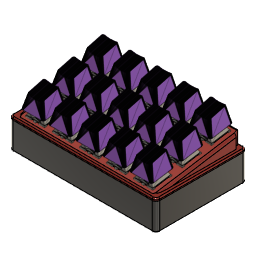
BFDeck x15 v4 (Autodesk Fusion 360 design; units mm, degrees)
Autodesk Fusion 360 part; units mm, degrees
note: some values were not read from the file. Chosen so that the rebuilt part matches the saved one: a direction; which face or edge a step refers to; which pieces of a blend or face edit are solid. Set by a fixed rule: which sketch regions a step uses.
sketch "Sketch1" plane through (0, 0, 0) normal (0, 0, 1) x (1, 0, 0)
  line L0 (-28.1946, -17.8088) -> (89.8054, -17.8088)
  line L1 (89.8054, -17.8088) -> (89.8054, 55.1912)
  line L2 (89.8054, 55.1912) -> (-28.1946, 55.1912)
  line L3 (-28.1946, 55.1912) -> (-28.1946, -17.8088)
  line L4 (87.8054, 53.1912) -> (-26.1946, 53.1912)
  line L5 (-26.1946, 53.1912) -> (-26.1946, -15.8088)
  line L6 (-26.1946, -15.8088) -> (87.8054, -15.8088)
  line L7 (87.8054, -15.8088) -> (87.8054, 53.1912)
  line L8 (87.8054, 53.1912) -> (-26.1946, -15.8088) construction
  line L9 (-26.1946, 53.1912) -> (87.8054, -15.8088) construction
  point P0 (30.8054, 18.6912)
  dimension "d1" = 114
  dimension "d2" = 69
  dimension "d104" = 2
  dimension "d106" = 2
  dimension "d136" = 2
  dimension "d137" = 2
  constraint horizontal L0
  constraint vertical L1
  constraint horizontal L2
  constraint vertical L3
  constraint horizontal L4
  constraint perpendicular L4 L5
  constraint parallel L4 L6
  constraint parallel L5 L7
  constraint coincident L8 P0
  constraint coincident L9 P0
  measures "d1" distance of L5.end L6.end
  measures "d2" distance of L4.end L5.end
  measures "d104" distance of L3 L5
  measures "d106" distance of L0 L6
  measures "d136" distance of L2 L4
  measures "d137" distance of L1 L7
extrude "Extrude1" add sketch "Sketch1" along normal blind 2 contours L0 L1 L2 L3 | L4 L5 L6 L7 makes body 1
sketch "Sketch2" plane through (0, 0, 2) normal (0, 0, 1) x (-1, 0, 0)
  line L0 (28.1946, -55.1912) -> (28.1946, 17.8088)
  line L1 (28.1946, 17.8088) -> (-89.8054, 17.8088)
  line L2 (-89.8054, 17.8088) -> (-89.8054, -55.1912)
  line L3 (-89.8054, -55.1912) -> (28.1946, -55.1912)
  line L4 (-87.8054, -53.1912) -> (26.1946, -53.1912)
  line L5 (26.1946, -53.1912) -> (26.1946, 15.8088)
  line L6 (26.1946, 15.8088) -> (-87.8054, 15.8088)
  line L7 (-87.8054, 15.8088) -> (-87.8054, -53.1912)
  line L8 (-87.8054, -53.1912) -> (26.1946, 15.8088) construction
  line L9 (26.1946, -53.1912) -> (-87.8054, 15.8088) construction
  point P0 (-30.8054, -18.6912)
  dimension "d7" = 114
  dimension "d8" = 69
  dimension "d107" = 2
  dimension "d108" = 2
  constraint horizontal L4
  constraint perpendicular L4 L5
  constraint parallel L4 L6
  constraint parallel L5 L7
  constraint coincident L8 P0
  constraint coincident L9 P0
  measures "d7" distance of L5.end L6.end
  measures "d8" distance of L4.start L6.end
  measures "d107" distance of L3 L4
  measures "d108" distance of L2 L7
extrude "Extrude2" add sketch "Sketch2" along normal blind 20 bodies 1
fillet "Fillet1" radius 3 1 edges at (89.8054, 55.1912, 11) on bodies 1
fillet "Fillet2" radius 3 3 edges at (-28.1946, 55.1912, 11) (-28.1946, -17.8088, 11) (89.8054, -17.8088, 11) on bodies 1
sketch "Sketch3" plane through (0, 0, 2) normal (0, 0, 1) x (-1, 0, 0)
  line L0 (-87.8054, -53.1912) -> (26.1946, -53.1912)
  line L1 (-87.8054, 15.8088) -> (-87.8054, -53.1912)
  line L2 (26.1946, -53.1912) -> (22.1946, -53.1912)
  line L3 (22.1946, -53.1912) -> (22.1946, -52.1912)
  line L4 (25.1946, -49.1912) -> (26.1946, -49.1912)
  line L5 (26.1946, -49.1912) -> (26.1946, -53.1912)
  arc A0 (25.1946, -49.1912) -> (22.1946, -52.1912) centre (25.1946, -52.1912) ccw
  circle A1 centre (25.1946, -52.1912) radius 1
  line L6 (-30.8054, -53.1912) -> (-30.8054, 38.8966)
  line L7 (59.5295, -18.6912) -> (-87.8054, -18.6912)
  line L8 (-87.8054, -49.1912) -> (-87.8054, -53.1912)
  circle A2 centre (-86.8054, -52.1912) radius 1
  arc A3 (-83.8054, -52.1912) -> (-86.8054, -49.1912) centre (-86.8054, -52.1912) ccw
  line L9 (-86.8054, -49.1912) -> (-87.8054, -49.1912)
  line L10 (-87.8054, -53.1912) -> (-83.8054, -53.1912)
  line L11 (-83.8054, -53.1912) -> (-83.8054, -52.1912)
  arc A4 (-86.8054, 11.8088) -> (-83.8054, 14.8088) centre (-86.8054, 14.8088) ccw
  line L12 (-86.8054, 11.8088) -> (-87.8054, 11.8088)
  line L13 (22.1946, 15.8088) -> (22.1946, 14.8088)
  line L14 (-87.8054, 15.8088) -> (26.1946, 15.8088)
  arc A5 (22.1946, 14.8088) -> (25.1946, 11.8088) centre (25.1946, 14.8088) ccw
  line L15 (26.1946, 15.8088) -> (22.1946, 15.8088)
  circle A6 centre (25.1946, 14.8088) radius 1
  line L16 (-83.8054, 15.8088) -> (-83.8054, 14.8088)
  line L17 (26.1946, 11.8088) -> (26.1946, 15.8088)
  line L18 (-87.8054, 11.8088) -> (-87.8054, 15.8088)
  line L19 (25.1946, 11.8088) -> (26.1946, 11.8088)
  circle A7 centre (-86.8054, 14.8088) radius 1
  line L20 (-87.8054, 15.8088) -> (-83.8054, 15.8088)
  line L21 (26.1946, -53.1912) -> (26.1946, 15.8088)
  line L22 (26.1946, 15.8088) -> (-87.8054, 15.8088)
  line L23 (87.2649, 1.901) -> (55, 1.901)
  line L24 (55, 1.901) -> (55, -5)
  line L25 (55, -5) -> (87.2649, -5)
  line L26 (87.2649, -5) -> (87.2649, 1.901)
  point P0 (22.1946, -49.1912)
  point P1 (-83.8054, -49.1912)
  point P2 (-87.8054, -53.1912)
  point P3 (-30.8054, 15.8088)
  point P4 (-87.8054, 15.8088)
  point P5 (22.1946, 11.8088)
  point P6 (-83.8054, 11.8088)
  dimension "d15" = 4
  dimension "d16" = 4
  dimension "d17" = 3
  dimension "d18" = 2
  constraint horizontal L2
  constraint vertical L3
  constraint horizontal L4
  constraint vertical L5
  constraint coincident L0.end L2.start
  constraint coincident P0 L3
  constraint coincident P0 L4
  constraint tangent L3 A0
  constraint tangent L4 A0
  constraint midpoint L0 L6.start
  constraint midpoint L1 L7.end
  constraint symmetric L0.end L6 L0.start
  constraint symmetric L0.end L6 P2
  constraint symmetric L2.end L6 L10.end
  constraint symmetric P0 L6 P1
  constraint symmetric L4.end L6 L8.start
  constraint symmetric L3.end L6 A3.start
  constraint symmetric L4.start L6 A3.end
  constraint symmetric A0 L6 A3
  constraint symmetric A1 L6 A2
  constraint symmetric P2 L7 P4
  constraint symmetric L0.end L7 L14.end
  constraint symmetric L2.end L7 L13.start
  constraint symmetric P0 L7 P5
  constraint symmetric L4.end L7 L17.start
  constraint symmetric L3.end L7 L13.end
  constraint symmetric L4.start L7 A5.end
  constraint symmetric A0 L7 A5
  constraint symmetric A1 L7 A6
  constraint symmetric L6.start L7 P3
  constraint symmetric L7 P1 P6
  constraint symmetric L7 P2 P4
  constraint symmetric L7 L10.end L16.start
  constraint symmetric L7 A3.end A4.start
  constraint symmetric L7 A3.start A4.end
  constraint symmetric L7 L8.start L12.end
  constraint symmetric L7 A2 A7
  constraint symmetric L7 A3 A4
  constraint coincident A0.centre A1.centre
  constraint horizontal L23
  constraint vertical L24
  constraint horizontal L25
  constraint vertical L26
  constraint parallel L7 L25
  constraint parallel L6 L24
  measures "d15" distance of L0.end L2.end
  measures "d16" distance of L2.end P0
  measures "d17" radius of A0
  measures "d18" diameter of A1
extrude "Extrude3" add sketch "Sketch3" along normal blind 20 contours L0 L1 L8 A2 A3 L9 L10 L11 | L0 L1 L8 A2 L10 | L0 L2 L3 L4 L5 A0 A1 L21 | L0 L2 L5 A1 L21 | L1 A4 L12 L14 L16 L18 A7 L20 L22 | L13 L14 A5 L15 A6 L17 L19 L21 L22 | L1 L14 L18 A7 L20 L22 | L14 L15 A6 L17 L21 L22 bodies 1
fillet "Fillet3" radius 1 8 edges at (30.8054, 55.1912, 0) (-27.316, 54.3125, 0) (-28.1946, 18.6912, 0) (-27.316, -16.9301, 0) (30.8054, -17.8088, 0) (88.9267, -16.9301, 0) (89.8054, 18.6912, 0) (88.9267, 54.3125, 0) on bodies 1
sketch "Sketch1 (2)" plane through (0, 0, 22) normal (0, 0, 1) x (-1, 0, 0) in component "Component"
  line L0 (22.1946, -53.1912) -> (-83.8054, -53.1912)
  line L1 (-87.8054, -49.1912) -> (-87.8054, 11.8088)
  line L2 (26.1946, -49.1912) -> (25.1946, -49.1912)
  arc A0 (25.1946, -49.1912) -> (22.1946, -52.1912) centre (25.1946, -52.1912) ccw
  line L3 (22.1946, -52.1912) -> (22.1946, -53.1912)
  circle A1 centre (25.1946, -52.1912) radius 1
  arc A2 (-86.8054, 17.8088) -> (-89.8054, 14.8088) centre (-86.8054, 14.8088) ccw
  line L4 (-89.8054, 14.8088) -> (-89.8054, -52.1912)
  arc A3 (-89.8054, -52.1912) -> (-86.8054, -55.1912) centre (-86.8054, -52.1912) ccw
  line L5 (-86.8054, -55.1912) -> (25.1946, -55.1912)
  arc A4 (25.1946, -55.1912) -> (28.1946, -52.1912) centre (25.1946, -52.1912) ccw
  line L6 (25.1946, -55.1912) -> (-86.8054, -55.1912)
  line L7 (-89.8054, -52.1912) -> (-89.8054, 14.8088)
  line L8 (-86.8054, 17.8088) -> (25.1946, 17.8088)
  line L9 (28.1946, 14.8088) -> (28.1946, -52.1912)
  arc A5 (28.1946, 14.8088) -> (25.1946, 17.8088) centre (25.1946, 14.8088) ccw
  arc A6 (25.1946, -55.1912) -> (28.1946, -52.1912) centre (25.1946, -52.1912) ccw
  arc A7 (-89.8054, -52.1912) -> (-86.8054, -55.1912) centre (-86.8054, -52.1912) ccw
  arc A8 (-86.8054, 17.8088) -> (-89.8054, 14.8088) centre (-86.8054, 14.8088) ccw
  line L10 (-83.8054, 15.8088) -> (22.1946, 15.8088)
  line L11 (26.1946, 11.8088) -> (26.1946, -49.1912)
  line L12 (28.1946, -52.1912) -> (28.1946, 14.8088)
  arc A9 (28.1946, 14.8088) -> (25.1946, 17.8088) centre (25.1946, 14.8088) ccw
  line L13 (25.1946, 17.8088) -> (-86.8054, 17.8088)
  line L14 (-83.8054, -53.1912) -> (-83.8054, -52.1912)
  arc A10 (-83.8054, -52.1912) -> (-86.8054, -49.1912) centre (-86.8054, -52.1912) ccw
  line L15 (-86.8054, -49.1912) -> (-87.8054, -49.1912)
  line L16 (-87.8054, 11.8088) -> (-86.8054, 11.8088)
  arc A11 (-86.8054, 11.8088) -> (-83.8054, 14.8088) centre (-86.8054, 14.8088) ccw
  line L17 (-83.8054, 14.8088) -> (-83.8054, 15.8088)
  line L18 (22.1946, 15.8088) -> (22.1946, 14.8088)
  arc A12 (22.1946, 14.8088) -> (25.1946, 11.8088) centre (25.1946, 14.8088) ccw
  line L19 (25.1946, 11.8088) -> (26.1946, 11.8088)
  circle A13 centre (-86.8054, -52.1912) radius 1
  circle A14 centre (-86.8054, 14.8088) radius 1
  circle A15 centre (25.1946, 14.8088) radius 1
  point P0 (-72, -52)
  point P1 (-8, -52)
  point P2 (-72, -8)
  point P3 (-72, -52)
  point P4 (-8, -52)
  point P5 (-8, -8)
  point P6 (-72, -8)
  point P7 (-72, -52)
  point P8 (-8, -52)
  point P9 (-8, -8)
  point P10 (-72, -8)
  point P11 (-72, -52)
  point P12 (-8, -52)
  point P13 (-8, -8)
  point P14 (-72, -8)
  point P15 (-72, -52)
  point P16 (-8, -52)
  point P17 (-8, -8)
  point P18 (-72, -8)
  point P19 (-72, -52)
  point P20 (-8, -52)
  point P21 (-8, -8)
  point P22 (-71.8054, -8.1912)
  point P23 (-71.8054, -52.1912)
  point P24 (-7.8054, -52.1912)
  point P25 (-7.8054, -8.1912)
  point P26 (-71.8054, 37.8088)
  point P27 (-71.8054, -52.1912)
  point P28 (58.1946, -52.1912)
  point P29 (58.1946, 37.8088)
  point P30 (27.0231, -52.1912)
  point P31 (25.1946, -52.1912)
  point P32 (25.1946, 14.8088)
  point P33 (25.1946, -52.1912)
  point P34 (25.1946, 14.8088)
  dimension "d26" = 3
  constraint horizontal L6
  constraint vertical L7
  constraint horizontal L8
  constraint tangent L8 A5
  constraint tangent L9 A5
  constraint tangent L6 A6
  constraint tangent L9 A6
  constraint equal A5 A6
  constraint tangent L6 A7
  constraint tangent L7 A7
  constraint equal A5 A7
  constraint tangent L7 A8
  constraint tangent L8 A8
  constraint equal A5 A8
  constraint collinear L4 L7
  constraint collinear L5 L6
  constraint collinear L9 L12
  constraint collinear L8 L13
  measures "d26" radius of A5
extrude "Extrude1'" add sketch "Sketch1 (2)" along normal blind 2 separate body contours L0 L1 L2 A0 L3 L10 L11 L14 A10 L15 L16 A11 L17 L18 A12 L19 | A2 L4 A3 L5 A4 L6 L7 L8 L9 A5 A6 A7 A8 L12 A9 L13 | A13 | A14 | A15 makes body 2 in component "Component"
sketch "Sketch2 (2)" plane through (0, 0, 24) normal (0, 0, 1) x (-1, 0, 0) in component "Component"
  arc A0 (-86.8054, 17.8088) -> (-89.8054, 14.8088) centre (-86.8054, 14.8088) ccw
  line L0 (-89.8054, 14.8088) -> (-89.8054, -52.1912)
  arc A1 (-89.8054, -52.1912) -> (-86.8054, -55.1912) centre (-86.8054, -52.1912) ccw
  line L1 (-86.8054, -55.1912) -> (25.1946, -55.1912)
  arc A2 (25.1946, -55.1912) -> (28.1946, -52.1912) centre (25.1946, -52.1912) ccw
  circle A3 centre (25.1946, -52.1912) radius 2.5
  line L2 (-30.8054, -55.1912) -> (-30.8054, -1.309)
  line L3 (-4.7878, -18.6912) -> (-89.8054, -18.6912)
  circle A4 centre (-86.8054, -52.1912) radius 2.5
  circle A5 centre (25.1946, 14.8088) radius 2.5
  circle A6 centre (-86.8054, 14.8088) radius 2.5
  line L4 (25.1946, -53.1912) -> (-86.8054, -53.1912)
  line L5 (-86.8054, -53.1912) -> (-86.8054, 14.8088)
  line L6 (-86.8054, 14.8088) -> (25.1946, 14.8088)
  line L7 (25.1946, 14.8088) -> (25.1946, -53.1912)
  arc A7 (28.1946, 14.8088) -> (25.1946, 17.8088) centre (25.1946, 14.8088) ccw
  line L8 (25.1946, 17.8088) -> (-86.8054, 17.8088)
  line L9 (28.1946, -52.1912) -> (28.1946, 14.8088)
  circle A8 centre (25.1946, -52.1912) radius 1
  point P0 (-86.8054, -53.1912)
  dimension "d29" = 5
  constraint midpoint L1 L2.start
  constraint midpoint L0 L3.end
  constraint symmetric A3 L2 A4
  constraint symmetric A3 L3 A5
  constraint symmetric L3 A4 A6
  constraint horizontal L4
  constraint vertical L5
  constraint horizontal L6
  constraint vertical L7
  constraint coincident L4 P0
  constraint parallel L3 L8
  constraint parallel L0 L2
  constraint coincident A5.centre L6.end
  constraint coincident A0.centre A6.centre
  measures "d29" diameter of A3
extrude "Extrude2'" add sketch "Sketch2 (2)" along normal blind 14 contours A3 L2 L3 A5 A6 L4 L5 L6 L7 | L2 L3 A4 L4 L5 bodies 2 in component "Component"
sketch "Sketch5" plane through (86.8054, 0, 0) normal (1, 0, 0) x (0, 1, 0)
  line L0 (-12.3088, 24) -> (49.6912, 24)
  line L1 (49.6912, 38) -> (-12.3088, 38)
  line L2 (49.6912, 24) -> (49.6912, 38)
  line L3 (-12.3088, 38) -> (-12.3088, 24)
sketch "Sketch6" plane through (86.8054, 0, 0) normal (1, 0, 0) x (0, 1, 0)
  line L0 (-14.8088, 24) -> (-14.8088, 38)
  line L1 (-14.8088, 24) -> (52.1912, 24)
  line L2 (-14.8088, 24) -> (52.4981, 34.599)
  line L3 (49.6912, 38) -> (53.1912, 38)
  line L4 (-14.8088, 24) -> (-14.8088, 38)
  line L5 (-14.8088, 38) -> (52.754, 38)
  line L6 (52.4981, 34.599) -> (55.5416, 34.599)
  line L7 (55.5416, 34.599) -> (55.5416, 38)
  line L8 (55.5416, 38) -> (46.6469, 38)
  dimension "d143" = 8.949
  constraint coincident L5.end L3
  constraint coincident L0.end L4.end
  constraint coincident L0.start L1.start
  constraint horizontal L6
  constraint perpendicular L3 L7
  constraint coincident L5 L8.end
  constraint perpendicular L7 L8
  measures "d143" angle of L1 L2
extrude "Extrude4" cut sketch "Sketch6" against normal blind 178 bodies 2 in component "Component"
fillet "Fillet1'" radius 1.883 4 edges at (86.8054, 18.6912, 29.2753) (-25.1946, 18.6912, 29.2753) (86.8054, -12.3088, 24.1968) (-25.1946, -12.3088, 24.1968) on bodies 2 in component "Component"
fillet "Fillet2'" radius 1 9 edges at (88.9267, -16.9301, 24) (89.8054, 18.6912, 24) (88.9267, 54.3125, 24) (30.8054, 55.1912, 24) (-27.316, 54.3125, 24) (-28.1946, 18.6912, 24) (-27.316, -16.9301, 24) (30.8054, -17.8088, 24) (88.9267, -16.9301, 24) on bodies 2 in component "Component"
sketch "Sketch7" plane through (0, -4.0462, 25.6948) normal (0, -0.155556, 0.987827) x (1, 0, 0)
  line L0 (84.9224, -9.2305) -> (84.9224, 55.2657)
  line L1 (-23.3116, 55.2657) -> (-23.3116, -9.2305)
  ellipse E0 centre (71.8054, -33.9372) end of major axis (71.8054, -31.4084) minor radius 2.5 (70.3683, -31.8679) -> (69.5942, -32.7573) ccw
  line L2 (8.1343, -33.3219) -> (70.3683, -33.3219)
  ellipse E1 centre (-58.1946, -33.9372) end of major axis (-58.1946, -31.4084) minor radius 2.5 (-55.9834, -32.7573) -> (-56.6535, -31.946) ccw
  line L3 (69.5942, -32.7573) -> (-55.9834, -32.7573)
  line L4 (-19.5142, 53.9919) -> (-5.5142, 53.9919)
  line L5 (-5.5142, 53.9919) -> (-5.5142, 39.9919)
  line L6 (-5.5142, 39.9919) -> (-19.5142, 39.9919)
  line L7 (-19.5142, 39.9919) -> (-19.5142, 53.9919)
  line L8 (2.2358, 53.9919) -> (16.2358, 53.9919)
  line L9 (2.2358, 39.9919) -> (2.2358, 53.9919)
  line L10 (16.2358, 39.9919) -> (2.2358, 39.9919)
  line L11 (16.2358, 53.9919) -> (16.2358, 39.9919)
  line L12 (23.9858, 53.9919) -> (37.9858, 53.9919)
  line L13 (23.9858, 39.9919) -> (23.9858, 53.9919)
  line L14 (37.9858, 39.9919) -> (23.9858, 39.9919)
  line L15 (37.9858, 53.9919) -> (37.9858, 39.9919)
  line L16 (45.7358, 53.9919) -> (59.7358, 53.9919)
  line L17 (45.7358, 39.9919) -> (45.7358, 53.9919)
  line L18 (59.7358, 39.9919) -> (45.7358, 39.9919)
  line L19 (59.7358, 53.9919) -> (59.7358, 39.9919)
  line L20 (67.4858, 53.9919) -> (81.4858, 53.9919)
  line L21 (67.4858, 39.9919) -> (67.4858, 53.9919)
  line L22 (81.4858, 39.9919) -> (67.4858, 39.9919)
  line L23 (81.4858, 53.9919) -> (81.4858, 39.9919)
  line L24 (-19.5142, 29.9919) -> (-5.5142, 29.9919)
  line L25 (-19.5142, 15.9919) -> (-19.5142, 29.9919)
  line L26 (-5.5142, 15.9919) -> (-19.5142, 15.9919)
  line L27 (-5.5142, 29.9919) -> (-5.5142, 15.9919)
  line L28 (2.2358, 29.9919) -> (16.2358, 29.9919)
  line L29 (2.2358, 15.9919) -> (2.2358, 29.9919)
  line L30 (16.2358, 15.9919) -> (2.2358, 15.9919)
  line L31 (16.2358, 29.9919) -> (16.2358, 15.9919)
  line L32 (23.9858, 29.9919) -> (37.9858, 29.9919)
  line L33 (23.9858, 15.9919) -> (23.9858, 29.9919)
  line L34 (37.9858, 15.9919) -> (23.9858, 15.9919)
  line L35 (37.9858, 29.9919) -> (37.9858, 15.9919)
  line L36 (45.7358, 29.9919) -> (59.7358, 29.9919)
  line L37 (45.7358, 15.9919) -> (45.7358, 29.9919)
  line L38 (59.7358, 15.9919) -> (45.7358, 15.9919)
  line L39 (59.7358, 29.9919) -> (59.7358, 15.9919)
  line L40 (67.4858, 29.9919) -> (81.4858, 29.9919)
  line L41 (67.4858, 15.9919) -> (67.4858, 29.9919)
  line L42 (81.4858, 15.9919) -> (67.4858, 15.9919)
  line L43 (81.4858, 29.9919) -> (81.4858, 15.9919)
  line L44 (-19.5142, 5.9919) -> (-5.5142, 5.9919)
  line L45 (-19.5142, -8.0081) -> (-19.5142, 5.9919)
  line L46 (-5.5142, -8.0081) -> (-19.5142, -8.0081)
  line L47 (-5.5142, 5.9919) -> (-5.5142, -8.0081)
  line L48 (2.2358, 5.9919) -> (16.2358, 5.9919)
  line L49 (2.2358, -8.0081) -> (2.2358, 5.9919)
  line L50 (16.2358, -8.0081) -> (2.2358, -8.0081)
  line L51 (16.2358, 5.9919) -> (16.2358, -8.0081)
  line L52 (23.9858, 5.9919) -> (37.9858, 5.9919)
  line L53 (23.9858, -8.0081) -> (23.9858, 5.9919)
  line L54 (37.9858, -8.0081) -> (23.9858, -8.0081)
  line L55 (37.9858, 5.9919) -> (37.9858, -8.0081)
  line L56 (45.7358, 5.9919) -> (59.7358, 5.9919)
  line L57 (45.7358, -8.0081) -> (45.7358, 5.9919)
  line L58 (59.7358, -8.0081) -> (45.7358, -8.0081)
  line L59 (59.7358, 5.9919) -> (59.7358, -8.0081)
  line L60 (67.4858, 5.9919) -> (81.4858, 5.9919)
  line L61 (67.4858, -8.0081) -> (67.4858, 5.9919)
  line L62 (81.4858, -8.0081) -> (67.4858, -8.0081)
  line L63 (81.4858, 5.9919) -> (81.4858, -8.0081)
  ellipse E2 centre (-25.1946, -10.8952) end of major axis (-25.1946, -13.426) minor radius 2.5 (-22.6946, -10.8952) -> (-23.3116, -9.2305) ccw
  line L64 (-22.6946, -10.8952) -> (84.3054, -10.8952)
  ellipse E3 centre (-25.1946, 56.9304) end of major axis (-25.1946, 54.3996) minor radius 2.5 (-23.3116, 55.2657) -> (-22.7136, 57.2411) ccw
  ellipse E4 centre (86.8054, -10.8952) end of major axis (86.8054, -13.426) minor radius 2.5 (84.9224, -9.2305) -> (84.3054, -10.8952) ccw
  ellipse E5 centre (86.8054, 56.9304) end of major axis (86.8054, 54.3996) minor radius 2.5 (84.3243, 57.2411) -> (84.9224, 55.2657) ccw
  line L65 (84.3243, 57.2411) -> (-22.7136, 57.2411)
  point P0 (39.2513, -33.3219)
  dimension "d116" = 14
  dimension "d117" = 14
  dimension "d120" = 87
  dimension "d121" = -48
  constraint horizontal L4
  constraint vertical L5
  constraint horizontal L6
  constraint vertical L7
  measures "d116" distance of L4.start L6.end
  measures "d117" distance of L4.start L4.end
extrude "Extrude8" cut sketch "Sketch7" against normal blind 30 contours L4 L5 L6 L7 | L8 L9 L10 L11 | L12 L13 L14 L15 | L16 L17 L18 L19 | L20 L21 L22 L23 | L24 L25 L26 L27 | L28 L29 L30 L31 | L32 L33 L34 L35 | L36 L37 L38 L39 | L40 L41 L42 L43 | L44 L45 L46 L47 | L48 L49 L50 L51 | L52 L53 L54 L55 | L56 L57 L58 L59 | L60 L61 L62 L63 bodies 2 in component "Component"
ref_plane "WorkPlane5" through (0, 0, 39) normal (0, 0, 1) x (1, 0, 0)
sketch "Sketch19" plane through (0, 0, 39) normal (0, 0, 1) x (1, 0, 0)
sketch "Sketch20" plane through (-25.1946, 0, 0) normal (-1, 0, 0) x (0, -1, 0)
  line L0 (2.7038, 24) -> (-49.6912, 32.2508)
  line L1 (-49.6912, 32.2508) -> (-49.6912, 24)
  line L2 (-49.6912, 24) -> (2.7038, 24)
ref_plane "WorkPlane1" through (30.8054, 21.178, 14.4821) normal (0, -0.155556, 0.987827) x (0, 0.987827, 0.155556)
sketch "Sketch11" plane through (0, 55.1912, 0) normal (0, 1, 0) x (-1, 0, 0)
  line L0 (-86.8054, 1) -> (25.1946, 1)
  line L1 (25.1946, 1) -> (25.1946, 22)
  line L2 (25.1946, 22) -> (-86.8054, 22)
  line L3 (-86.8054, 22) -> (-86.8054, 1)
  line L4 (-86.8054, 22) -> (25.1946, 22)
  line L5 (25.1946, 22) -> (25.1946, 1)
  line L6 (25.1946, 1) -> (-86.8054, 1)
  line L7 (-86.8054, 1) -> (-86.8054, 22)
  line L8 (-34.8054, 6) -> (-26.8054, 6)
  line L9 (-34.8054, 3) -> (-34.8054, 6)
  line L10 (-26.8054, 3) -> (-34.8054, 3)
  line L11 (-26.8054, 6) -> (-26.8054, 3)
  line L12 (-86.8054, 1) -> (25.1946, 1)
  line L13 (-30.8054, 7) -> (-30.8054, -5)
  dimension "d90" = 3
  dimension "d91" = 8
  dimension "d145" = 2
  constraint horizontal L4
  constraint vertical L5
  constraint horizontal L6
  constraint vertical L7
  constraint coincident L0.end L1.start
  constraint coincident L2.end L3.start
  constraint horizontal L8
  constraint vertical L11
  constraint horizontal L10
  constraint vertical L9
  constraint coincident L0.start L3.end
  constraint perpendicular L6 L13
  constraint midpoint L6 L13
  constraint symmetric L9 L11 L13
  measures "d90" distance of L10.start L8.end
  measures "d91" distance of L8.end L8.start
  measures "d145" distance of L6 L10
extrude "Extrude5" cut sketch "Sketch11" against normal blind 13 contours L8 L9 L10 L13 | L8 L10 L11 L13 bodies 1
sketch "Sketch12" plane through (0, 53.1912, 0) normal (0, -1, 0) x (1, 0, 0)
  line L0 (-22.1946, 22) -> (-22.1946, 2)
  line L1 (83.8054, 22) -> (-22.1946, 22)
  line L2 (26.8054, 6) -> (34.8054, 6)
  line L3 (50.8054, 2) -> (10.8054, 2)
  line L4 (10.8054, 2) -> (10.8054, 3.5)
  line L5 (10.8054, 3.5) -> (50.8054, 3.5)
  line L6 (50.8054, 3.5) -> (50.8054, 2)
  line L7 (50.8054, 2) -> (10.8054, 3.5) construction
  line L8 (10.8054, 2) -> (50.8054, 3.5) construction
  line L9 (83.8054, 2) -> (83.8054, 22)
  line L10 (83.8054, 2) -> (-22.1946, 2)
  point P0 (30.8054, 2.75)
  dimension "d146" = 40
  dimension "d147" = 1.5
  constraint horizontal L3
  constraint perpendicular L3 L4
  constraint parallel L3 L5
  constraint parallel L4 L6
  constraint coincident L7 P0
  constraint coincident L8 P0
  constraint collinear L3 L10
  constraint midpoint L3 L10
  measures "d146" distance of L4.end L5.end
  measures "d147" distance of L3.end L4.end
extrude "Extrude6" cut sketch "Sketch12" against normal blind 1.5 contours L3 L4 L5 L6 L10 bodies 1
other "Base Mesh Feature1"
other "Modify1"
other "Modify2"
other "CopyPasteMeshes1"
other "Modify3"
other "CopyPasteMeshes2"
other "Modify4"
sketch "Sketch15" plane through (0, 0, 0) normal (0, 1, 0) x (1, 0, 0)
ref_plane "WorkPlane3" through (0, 19, 0) normal (0, 1, 0) x (0, 0, 1)
sketch "Sketch16" plane through (0, 19, 0) normal (0, 1, 0) x (1, 0, 0)
sketch "Sketch17" plane through (0, 0, 0) normal (0, 0, 1) x (1, 0, 0)
ref_plane "WorkPlane4" through (30.8054, 17.4446, 38.1899) normal (0, -0.155556, 0.987827) x (0, 0.987827, 0.155556)
sketch "Sketch18" plane through (30.8054, 17.4446, 38.1899) normal (0, -0.155556, 0.987827) x (0, 0.987827, 0.155556)
other "Base Mesh Feature3"
other "Modify26"
other "Modify27"
other "Modify28"
ref_plane "WorkPlane7" through (30.8054, 21.2274, 14.168) normal (0, -0.155556, 0.987827) x (0, 0.987827, 0.155556)
sketch "Sketch22" plane through (30.8054, 21.2274, 14.168) normal (0, -0.155556, 0.987827) x (0, 0.987827, 0.155556)
  line L0 (-0.3109, -52.2105) -> (-0.3109, 52.7895)
  line L1 (-0.3109, 52.7895) -> (-0.3109, -52.2105)
  line L2 (32.6891, 0.2895) -> (-33.3109, 0.2895)
  line L3 (-33.3109, -52.2105) -> (32.6891, -52.2105)
  line L4 (32.6891, -52.2105) -> (32.6891, 52.7895)
  line L5 (32.6891, 52.7895) -> (-33.3109, 52.7895)
  line L6 (-33.3109, 52.7895) -> (-33.3109, -52.2105)
  line L7 (-33.3109, -52.2105) -> (32.6891, 52.7895) construction
  line L8 (32.6891, -52.2105) -> (-33.3109, 52.7895) construction
  point P0 (-0.3109, 0.2895)
  dimension "d140" = 105
  dimension "d141" = 66
  constraint vertical L0
  constraint vertical L1
  constraint horizontal L2
  constraint midpoint L1 L2
  constraint midpoint L0 L1
  constraint horizontal L3
  constraint perpendicular L3 L4
  constraint parallel L3 L5
  constraint parallel L4 L6
  constraint coincident L7 P0
  constraint coincident L8 P0
  constraint midpoint L1 P0
  constraint coincident L0.start L3
  constraint coincident L2.end L6
  measures "d140" distance of L0.end L0.start
  measures "d141" distance of L2.start L2.end
extrude "Extrude10" cut sketch "Sketch22" along normal blind 13.224 bodies 2 in component "Component"
other "CopyPasteMeshes12"
other "Modify29"
other "CopyPasteMeshes13"
other "Modify30"
ref_plane "WorkPlane8" through (30.8054, 18.8446, 29.2995) normal (0, -0.155556, 0.987827) x (0, 0.987827, 0.155556)
other "Modify51"
other "Modify52"
other "Modify53"
other "Modify54"
other "Modify55"
other "Modify56"
other "Modify57"
other "CopyPasteMeshes25"
other "Modify58"
other "CopyPasteMeshes26"
other "Modify59"
other "Modify60"
other "CopyPasteMeshes27"
other "Modify61"
other "Modify62"
component "Component" placed x (1, 0, 0) y (0, 1, 0) z (0, 0, 1) at (0, 0, 0)
equation "d2 = 92 mm * 0.75"
equation "d8 = 92 mm * 0.75"
equation "d129 = -15.148 mm - 0.17 mm"
